Autodesk Inventor part; units mm, degrees
(part 2 of 2)
  spline S107 degree 2 poles (-18.318, 92.5798) (-18.5205, 92.3897) (-18.8811, 92.0364) (-19.054, 91.8463) knots 0 0 0 1 2 2 2
  spline S108 degree 2 poles (-19.054, 91.8463) (-19.4023, 91.4634) (-19.6567, 91.004) (-19.6567, 90.7594) knots 0 0 0 1 2 2 2
  spline S109 degree 2 poles (-19.6567, 90.7594) (-19.6567, 90.631) (-19.5777, 90.4383) (-19.5061, 90.3766) knots 0 0 0 1 2 2 2
  spline S110 degree 2 poles (-19.5061, 90.3766) (-19.4344, 90.3148) (-19.2467, 90.2531) (-19.1331, 90.2531) knots 0 0 0 1 2 2 2
  spline S111 degree 2 poles (-19.1331, 90.2531) (-19.0244, 90.2531) (-18.8021, 90.3074) (-18.7008, 90.3494) knots 0 0 0 1 2 2 2
  spline S112 degree 2 poles (-18.7008, 90.3494) (-18.6144, 90.384) (-18.4538, 90.4828) (-18.4044, 90.5174) knots 0 0 0 1 2 2 2
  line L154 (-18.4044, 90.5174) -> (-18.3822, 90.5174)
  line L155 (-18.3822, 90.5174) -> (-18.3822, 90.0827)
  spline S113 degree 2 poles (-18.3822, 90.0827) (-18.5082, 90.0209) (-18.9602, 89.8999) (-19.1627, 89.8999) knots 0 0 0 1 2 2 2
  spline S114 degree 2 poles (-19.1627, 89.8999) (-19.59, 89.8999) (-20.0717, 90.3519) (-20.0717, 90.7372) knots 0 0 0 1 2 2 2
  spline S115 degree 2 poles (-20.0717, 90.7372) (-20.0717, 90.9175) (-19.9877, 91.2189) (-19.9136, 91.3473) knots 0 0 0 1 2 2 2
  spline S116 degree 2 poles (-19.9136, 91.3473) (-19.8395, 91.4807) (-19.6246, 91.7425) (-19.5061, 91.8685) knots 0 0 0 1 2 2 2
  spline S117 degree 2 poles (-19.5061, 91.8685) (-19.3134, 92.0784) (-18.8416, 92.528) (-18.7008, 92.6589) knots 0 0 0 1 2 2 2
  line L156 (-18.7008, 92.6589) -> (-20.1977, 92.6589)
  line L157 (-20.1977, 92.6589) -> (-20.1977, 93.0121)
  spline S118 degree 2 poles (-22.4528, 92.0439) (-22.4528, 92.2637) (-22.312, 92.6391) (-22.1836, 92.7774) knots 0 0 0 1 2 2 2
  spline S119 degree 2 poles (-22.1836, 92.7774) (-22.0551, 92.9158) (-21.6723, 93.0763) (-21.4351, 93.0763) knots 0 0 0 1 2 2 2
  spline S120 degree 2 poles (-21.4351, 93.0763) (-21.2178, 93.0763) (-20.7929, 92.98) (-20.6373, 92.9034) knots 0 0 0 1 2 2 2
  line L158 (-20.6373, 92.9034) -> (-20.6373, 92.4712)
  line L159 (-20.6373, 92.4712) -> (-20.667, 92.4712)
  spline S121 degree 2 poles (-20.667, 92.4712) (-20.7139, 92.5057) (-20.8893, 92.5947) (-20.9955, 92.6342) knots 0 0 0 1 2 2 2
  spline S122 degree 2 poles (-20.9955, 92.6342) (-21.1165, 92.6762) (-21.3166, 92.7231) (-21.4426, 92.7231) knots 0 0 0 1 2 2 2
  spline S123 degree 2 poles (-21.4426, 92.7231) (-21.5661, 92.7231) (-21.7982, 92.6342) (-21.8822, 92.5379) knots 0 0 0 1 2 2 2
  spline S124 degree 2 poles (-21.8822, 92.5379) (-21.9588, 92.4465) (-22.0378, 92.2044) (-22.0378, 92.0414) knots 0 0 0 1 2 2 2
  spline S125 degree 2 poles (-22.0378, 92.0414) (-22.0378, 91.8784) (-21.9489, 91.6709) (-21.8649, 91.6017) knots 0 0 0 1 2 2 2
  spline S126 degree 2 poles (-21.8649, 91.6017) (-21.7785, 91.5251) (-21.5216, 91.4609) (-21.366, 91.4609) knots 0 0 0 1 2 2 2
  spline S127 degree 2 poles (-21.366, 91.4609) (-21.198, 91.4609) (-20.8646, 91.5128) (-20.7633, 91.535) knots 0 0 0 1 2 2 2
  line L160 (-20.7633, 91.535) -> (-20.7633, 89.9641)
  line L161 (-20.7633, 89.9641) -> (-22.4355, 89.9641)
  line L162 (-22.4355, 89.9641) -> (-22.4355, 90.3222)
  line L163 (-22.4355, 90.3222) -> (-21.156, 90.3222)
  line L164 (-21.156, 90.3222) -> (-21.156, 91.1349)
  spline S128 degree 2 poles (-21.156, 91.1349) (-21.2301, 91.125) (-21.3734, 91.1176) (-21.4327, 91.1176) knots 0 0 0 1 2 2 2
  spline S129 degree 2 poles (-21.4327, 91.1176) (-21.6673, 91.1176) (-21.9909, 91.1942) (-22.1391, 91.3078) knots 0 0 0 1 2 2 2
  spline S130 degree 2 poles (-22.1391, 91.3078) (-22.2898, 91.4214) (-22.4528, 91.7672) (-22.4528, 92.0439) knots 0 0 0 1 2 2 2
  point P0 (-47.5, 53.2457)
  constraints: 2 other
extrude "Extrusion47" add sketch "Sketch58" along normal blind 1
sketch "Sketch59" plane through (69.5, 80.5, 0) normal (0, 0, -1) x (-1, 0, 0)
  line L0 (124.232, -148.2248) -> (124.232, -65.5994) projected
  line L1 (124.232, -131.7625) -> (22.225, -131.7625)
  line L2 (22.225, -144.4625) -> (124.232, -144.4625)
  line L3 (124.232, -144.4625) -> (124.232, -131.7625)
  line L4 (22.225, -144.4625) -> (19.05, -144.4625)
  line L5 (19.05, -144.4625) -> (19.05, -131.7625)
  line L6 (19.05, -131.7625) -> (22.225, -131.7625)
  point P0 (69.5, -80.5)
  point P1 (22.225, -131.7625)
  constraints: 12 end point, 2 horizontal, 2 parallel, 1 perpendicular, 1 point on line
extrude "Extrusion48" add sketch "Sketch59" against normal blind 1
sketch "Sketch61" plane through (-54.732, -66.7303, 5) normal (-1, 0, 0) x (0, 0, 1)
  point P0 (-5, 66.7303)
sketch "Sketch63" plane through (-54.732, -66.7303, 5) normal (-1, 0, 0) x (0, 0, 1)
  line L0 (0, 0) -> (32.8849, -46.9646) projected
  line L1 (32.8849, -46.9646) -> (72.2795, -19.3802)
  line L2 (72.2795, -19.3802) -> (86.4989, -39.6875)
  line L3 (86.4989, -39.6875) -> (32.8849, -46.9646)
  point P0 (-5, 66.7303)
  constraints: 6 end point, 2 perpendicular
extrude "Extrusion50" cut sketch "Sketch63" against normal blind 155.1
sketch "Sketch64" plane through (-54.732, -87.3593, 75.4961) normal (0, -0.819152, 0.5735764) x (1, 0, 0)
  line L0 (4, 0) -> (4, -5)
  line L1 (2, -5) -> (2, 0)
  line L2 (5, -5) -> (5, -6.5)
  line L3 (5, -6.5) -> (1, -6.5)
  line L4 (1, -6.5) -> (1, -5)
  line L5 (6, 0) -> (6, -45.9148) projected
  line L6 (1, -5) -> (2, -5)
  line L7 (4, -5) -> (5, -5)
  line L8 (2, 0) -> (2, 0.0793)
  line L9 (2, 0.0793) -> (4, 0.0793)
  line L10 (0, 0) -> (6, 0) projected
  line L11 (4, 0.0793) -> (4, 0)
  line L12 (0, -45.9148) -> (0, 21.0852) projected
  line L13 (100.464, 0) -> (100.464, -5)
  line L14 (102.464, -5) -> (102.464, 0)
  line L15 (99.464, -5) -> (99.464, -6.5)
  line L16 (99.464, -6.5) -> (103.464, -6.5)
  line L17 (103.464, -6.5) -> (103.464, -5)
  line L18 (103.464, -5) -> (102.464, -5)
  line L19 (100.464, -5) -> (99.464, -5)
  line L20 (102.464, 0.0793) -> (100.464, 0.0793)
  line L21 (102.464, 0) -> (102.464, 0.0793)
  line L22 (100.464, 0.0793) -> (100.464, 0)
  constraints: 40 end point, 5 parallel, 2 horizontal, 2 perpendicular, 1 collinear, 1 vertical
extrude "Extrusion51" cut sketch "Sketch64" against normal blind 100.765
body "Solid1"
